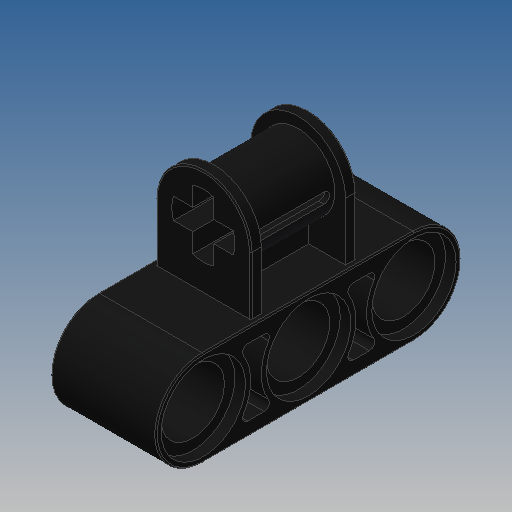
# Autodesk Inventor part: 63869-Black
Saved by Autodesk Inventor 2022.2 (Build 262287000, 287)
## iProperties
Created: 2014-07-08
Part Number: 63869-Black
Material: ABS Plastic
Document SubType Name: Modeling
Designer: D. Kohfeld
Mass: 0.893558 g
Surface Area: 15.5327 cm^2
Volume: 0.842979 cm^3
Density: 1.06 g/cm^3
Appearance: Black
Author: D. Kohfeld
Autodesk Inventor part; units mm, degrees
ref_plane "YZ Plane" through (0, 0, 0) normal (1, 0, 0) x (0, 1, 0)
ref_plane "XZ Plane" through (0, 0, 0) normal (0, 1, 0) x (-1, 0, 0)
ref_plane "XY Plane" through (0, 0, 0) normal (0, 0, 1) x (1, 0, 0)
sketch "Sketch2" plane through (0, 0, 0) normal (1, 0, 0) x (0, 1, 0)
  circle A0 centre (0, 8) radius 2.4
  circle A1 centre (0, 0) radius 2.4
  line L0 (0, 8) -> (0, 0) construction
  line L1 (0, 0) -> (0, -8) construction
  circle A2 centre (0, -8) radius 2.4
  line L2 (-3.6, 8) -> (-3.6, -8)
  arc A3 (-3.6, -8) -> (3.6, -8) centre (0, -8) ccw
  line L3 (3.6, -8) -> (3.6, 8)
  arc A4 (3.6, 8) -> (-3.6, 8) centre (0, 8) ccw
  dimension "d0" = 4.8
  dimension "d2" = 8
  dimension "d43" = 7.2
  constraints: 8 end point, 5 centre point, 4 point on circle, 4 tangent, 3 coincident, 2 collinear, 2 concentric, 2 equal radius, 2 parallel, 1 vertical
  measures "d0" diameter of A0
  measures "d2" distance of A1.centre L0.start
  measures "d43" diameter of A4
extrude "Extrusion1" add sketch "Sketch2" along normal mid plane 8
sketch "Sketch8" plane through (4, 0, 0) normal (1, 0, 0) x (0, 0, -1)
  circle A0 centre (8, 0) radius 2.4 projected
  circle A1 centre (0, 0) radius 2.4 projected
  circle A2 centre (-8, 0) radius 2.4 projected
  arc A3 (8, -3.6) -> (8, 3.6) centre (8, 0) ccw projected
  arc A4 (-8, 3.6) -> (-8, -3.6) centre (-8, 0) ccw projected
  circle A5 centre (-8, 0) radius 3.2
  circle A6 centre (0, 0) radius 3.2
  circle A7 centre (8, 0) radius 3.2
  line L0 (8, 3.6) -> (-8, 3.6) projected
  line L1 (-5.4544, 2.5456) -> (-2.5456, 2.5456)
  line L2 (-5.4544, -2.5456) -> (-2.5456, -2.5456)
  line L3 (2.5456, 2.5456) -> (5.4544, 2.5456)
  line L4 (2.5456, -2.5456) -> (5.4544, -2.5456)
  arc A8 (-5.4544, -2.5456) -> (-5.4544, 2.5456) centre (-8, 0) ccw
  arc A9 (-2.5456, 2.5456) -> (-2.5456, -2.5456) centre (0, 0) ccw
  arc A10 (2.5456, -2.5456) -> (2.5456, 2.5456) centre (0, 0) ccw
  arc A11 (5.4544, 2.5456) -> (5.4544, -2.5456) centre (8, 0) ccw
  line L5 (-8, 0) -> (-5.4544, 2.5456) construction
  dimension "d44" = 6.4
  dimension "d48" = 45
  constraints: 10 end point, 8 point on circle, 7 centre point, 7 coincident, 6 equal radius, 4 parallel, 3 equal length
  measures "d44" diameter of A5
  measures "d48" angle of L0 L5
extrude "Extrusion5" cut sketch "Sketch8" against normal blind 0.8 contours A5 | A6 | A7
extrude "Extrusion6" cut sketch "Sketch8" against normal blind 2.4 contours L1 A9 L2 A8 | L3 A11 L4 A10
mirror "Mirror2" about plane through (0, 0, 0) normal (1, 0, 0) of "Extrusion5", "Extrusion6"
sketch "Sketch4" plane through (0, 0, 0) normal (0, 0, 1) x (1, 0, 0)
  line L0 (-0.8, 3.6) -> (-0.8, 5.3167)
  line L1 (0.8, 3.6) -> (0.8, 5.3167)
  arc A0 (0.8, 5.3167) -> (-0.8, 5.3167) centre (0, 8) ccw
  circle A1 centre (0, 8) radius 2.4 construction
  line L2 (-0.8, 10.2627) -> (-0.8, 8.8)
  line L3 (-0.8, 8.8) -> (-2.2627, 8.8)
  line L4 (-2.2627, 7.2) -> (-0.8, 7.2)
  line L5 (-0.8, 7.2) -> (-0.8, 5.7373)
  line L6 (0.8, 5.7373) -> (0.8, 7.2)
  line L7 (0.8, 7.2) -> (2.2627, 7.2)
  line L8 (2.2627, 8.8) -> (0.8, 8.8)
  line L9 (0.8, 8.8) -> (0.8, 10.2627)
  arc A2 (0.8, 10.2627) -> (-0.8, 10.2627) centre (0, 8) ccw
  arc A3 (-2.2627, 8.8) -> (-2.2627, 7.2) centre (0, 8) ccw
  arc A4 (-0.8, 5.7373) -> (0.8, 5.7373) centre (0, 8) ccw
  arc A5 (2.2627, 7.2) -> (2.2627, 8.8) centre (0, 8) ccw
  line L10 (-4, 3.6) -> (4, 3.6) projected
  line L11 (-0.8, 3.6) -> (0.8, 3.6)
  point P0 (0, 0)
  dimension "d18" = 4.8
  dimension "d12" = 5.6
  dimension "d14" = 1.6
  dimension "d20" = 1.6
  dimension "d40" = 8
  constraints: 22 end point, 10 point on circle, 8 equal length, 5 centre point, 4 parallel, 4 perpendicular, 1 coincident, 1 collinear, 1 horizontal alignment, 1 point on line, 1 vertical, 1 vertical alignment, 14 other
  measures "d12" diameter of A0
  measures "d14" distance between parallel lines of L0 L1
  measures "d20" distance between parallel lines of L9 L2
  measures "d40" distance of A0.centre point (0, 0)
extrude "Extrusion2" add sketch "Sketch4" along normal mid plane 8
sketch "Sketch5" plane through (0, 0, 0) normal (1, 0, 0) x (0, 1, 0)
  line L0 (7.2, 4) -> (8.8, 4) projected
  line L1 (8.8, -4) -> (8.8, 4) projected
  line L2 (7.6, 2.4) -> (7.6, -2.4)
  arc A0 (7.6, -2.4) -> (8.4, -2.4) centre (8, -2.4) ccw
  line L3 (8.4, -2.4) -> (8.4, 2.4)
  arc A1 (8.4, 2.4) -> (7.6, 2.4) centre (8, 2.4) ccw
  point P0 (0, 0)
  point P1 (8, 4)
  point P2 (8.4, 0)
  point P3 (8.8, 0)
  dimension "d23" = 0.8
  dimension "d24" = 5.6
  constraints: 4 end point, 4 point on circle, 4 tangent, 3 midpoint, 2 centre point, 2 parallel, 1 horizontal alignment, 1 vertical alignment
  measures "d23" distance between parallel lines of L2 L3
extrude "Extrusion3" cut sketch "Sketch5" along normal through all both and the other way through all
sketch "Sketch6" plane through (0, 0, 4) normal (0, 0, 1) x (1, 0, 0)
  line L0 (3.6, 3.6) -> (3.6, 8)
  arc A0 (3.6, 8) -> (-3.6, 8) centre (0, 8) ccw
  line L1 (-3.6, 8) -> (-3.6, 3.6)
  arc A1 (0.8, 5.3167) -> (-0.8, 5.3167) centre (0, 8) ccw projected
  line L2 (-0.8, 5.3167) -> (-0.8, 3.6) projected
  line L3 (-0.8, 3.6) -> (-0.8, 5.3167)
  line L4 (0.8, 3.6) -> (0.8, 5.3167)
  arc A2 (0.8, 5.3167) -> (-0.8, 5.3167) centre (0, 8) ccw
  line L5 (0.8, 3.6) -> (0.8, 5.3167) projected
  line L6 (-3.6, 3.6) -> (-0.8, 3.6)
  line L7 (0.8, 3.6) -> (3.6, 3.6)
  dimension "d41" = 7.2
  constraints: 13 end point, 4 point on circle, 3 equal length, 3 tangent, 2 centre point, 2 perpendicular, 1 coincident, 1 vertical
  measures "d41" diameter of A0
extrude "Extrusion4" add sketch "Sketch6" against normal blind 0.8
mirror "Mirror1" about plane through (0, 0, 0) normal (0, 0, 1) of "Extrusion4"
fillet "Fillet1" radius 0.1 14 edges at (-3.6, 5.8, 4) (3.6, 5.8, 4) (0, 11.6, 4) (-3.6, 5.8, -4) (3.6, 5.8, -4) (0, 11.6, -4) (-4, 0, -11.6) (-4, -3.6, 0) (-4, 0, 11.6) (-4, 3.6, 0) (4, 0, 11.6) (4, -3.6, 0) (4, 0, -11.6) (4, 3.6, 0)
fillet "Fillet1" radius 0.4 16 edges at (2.8, 2.5456, 5.4544) (2.8, 2.5456, 2.5456) (2.8, 2.5456, -2.5456) (2.8, 2.5456, -5.4544) (2.8, -2.5456, 5.4544) (2.8, -2.5456, 2.5456) (2.8, -2.5456, -2.5456) (2.8, -2.5456, -5.4544) (-2.8, 2.5456, 2.5456) (-2.8, 2.5456, 5.4544) (-2.8, -2.5456, 5.4544) (-2.8, -2.5456, 2.5456) (-2.8, 2.5456, -2.5456) (-2.8, 2.5456, -5.4544) (-2.8, -2.5456, -2.5456) (-2.8, -2.5456, -5.4544)
equation "\"d0\" = tpd"
equation "\"d2\" = lu"
equation "\"d43\" = tlad"
equation "\"d3\" = lu"
equation "\"d44\" = tsd"
equation "\"d45\" = tsl"
equation "\"d18\" = kd"
equation "\"d14\" = wall"
equation "\"d20\" = axlet"
equation "\"d40\" = lu"
equation "\"d21\" = lu"
equation "\"d23\" = tpnw"
equation "\"d41\" = tlad"
equation "\"d29\" = tsl"
equation "\"d39\" = lf"
equation "\"d51\" = tf"
equation "\"tpd\" = 4.8"
equation "\"lu\" = 8"
equation "\"tlad\" = 7.2"
equation "\"tsd\" = 6.4"
equation "\"tsl\" = 0.8"
equation "\"kd\" = 4.8"
equation "\"wall\" = 1.6"
equation "\"axlet\" = 1.6"
equation "\"tpnw\" = 0.8"
equation "\"lf\" = 0.1"
equation "\"tf\" = 0.4"
body "Solid1"
